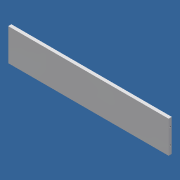
# Autodesk Inventor part: J001394
Saved by Autodesk Inventor 2012 SP2 (Build 160219200, 219)
## iProperties
Created: 2012-06-05
Part Number: J001394
Material: ALUMINUM, 6061-T651
Vendor: HHMI: JFRC - ID&F
Document SubType Name: Modeling
Designer: NEGRASHOVI
Density: 2.7 g/cm^3
Project: P-51601
Mass: 176.063 g
Surface Area: 294.127 cm^2
Volume: 65.2084 cm^3
Description: SIDE PANEL
RuleStatus: InUse
AfterDocSave0: file://Part Number Cleaner
LAB/DEPT: GONEN (LAB)
REQUESTING SCIENTIST: GONEN, TAMIR
SURFACE ROUGHNESS: 32 Ra
DESIGN DEPARTMENT: HHMI: JFRC - ID&F
SPECIAL FINISH: ANODIZE PER MIL-A-8625F, TYPE II, CLASS 2 (BLACK)
ALTERED ITEM PART NUMBER: N/A
ALTERED ITEM VENDOR: N/A
ALTERED ITEM DESCRIPTION: N/A
Author: NEGRASHOVI
Revision Number: -
Autodesk Inventor part; units mm, degrees
ref_plane "YZ Plane" through (0, 0, 0) normal (1, 0, 0) x (0, 1, 0)
ref_plane "XZ Plane" through (0, 0, 0) normal (0, 1, 0) x (-1, 0, 0)
ref_plane "XY Plane" through (0, 0, 0) normal (0, 0, 1) x (1, 0, 0)
sketch "Sketch1" plane through (0, 0, 0) normal (0, 0, 1) x (1, 0, 0)
  line L0 (-127, 25.4) -> (127, 25.4)
  line L1 (127, 25.4) -> (127, -25.4)
  line L2 (127, -25.4) -> (-127, -25.4)
  line L3 (-127, -25.4) -> (-127, 25.4)
  point P0 (0, 0)
  dimension "d0" = 254
  dimension "d1" = 50.8
  dimension "d2" = 25.4
  dimension "d3" = 127
  constraints: 8 end point, 2 parallel, 1 horizontal, 1 perpendicular
  measures "d0" distance of L0.start L0.end
  measures "d1" distance of L2.end L0.start
  measures "d2" distance from line of point (0, 0) L0
  measures "d3" distance from line of point (0, 0) L3
extrude "Extrusion1" add sketch "Sketch1" along normal blind 5.08
sketch "Sketch2" plane through (127, -25.4, 0) normal (1, 0, 0) x (0, 0, -1)
  line L0 (-5.08, 50.8) -> (-5.08, 0) projected
  line L1 (0, 0) -> (-5.08, 0) projected
  line L2 (0, 50.8) -> (0, 0) projected
  line L3 (0, 50.8) -> (-5.08, 50.8) projected
  line L4 (-2.54, 50.8) -> (-2.54, 0) construction
  line L5 (1.016, 25.4) -> (-6.096, 25.4) construction
  point P0 (0, 25.4)
  point P1 (-2.54, 38.1)
  point P2 (-2.54, 12.7)
  dimension "d6" = 25.4
  constraints: 2 end point, 2 midpoint, 2 point on line, 1 symmetric about line
  measures "d6" distance of point (-2.54, 38.1) point (-2.54, 12.7)
hole "Hole1" at (127, 12.7, 2.54) at (127, -12.7, 2.54) direction (-1, 0, 0) diameter 2.6416 depth 15.24 tip angle 118 thread size "6-32 UNC" class "2B" standard "ANSI Unified Screw Threads"
mirror "Mirror1" about plane through (0, 0, 0) normal (1, 0, 0) of "Hole1"
equation "\"d2\" = 0.5 * d1"
equation "\"d3\" = 0.5 * d0"
body "Solid1"
